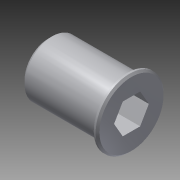
# Autodesk Inventor part: colson hub
Saved by Autodesk Inventor 2013 (Build 170138000, 138)
## iProperties
Created: 2012-09-06
Part Number: colson hub
Material: Aluminum 6061
Document SubType Name: Modeling
Designer: student
Density: 2.71 g/cm^3
Mass: 25.8237 g
Surface Area: 50.2015 cm^2
Volume: 9.52906 cm^3
Author: student
Autodesk Inventor part; units mm, degrees
ref_plane "YZ Plane" through (0, 0, 0) normal (1, 0, 0) x (0, 1, 0)
ref_plane "XZ Plane" through (0, 0, 0) normal (0, 1, 0) x (-1, 0, 0)
ref_plane "XY Plane" through (0, 0, 0) normal (0, 0, 1) x (1, 0, 0)
sketch "Sketch1" plane through (0, 0, 0) normal (1, 0, 0) x (0, 1, 0)
  circle A0 centre (0, 0) radius 11.684
  dimension "d0" = 23.368
  constraints: 1 centre point, 1 coincident
  measures "d0" diameter of A0
extrude "Extrusion1" add sketch "Sketch1" along normal blind 33.3375
sketch "Sketch2" plane through (33.3375, 0, 0) normal (1, 0, 0) x (0, 0, -1)
  circle A0 centre (0, 0) radius 11.684 projected
  circle A1 centre (0, 0) radius 14.2875
  dimension "d4" = 28.575
  constraints: 1 centre point, 1 coincident
  measures "d4" diameter of A1
extrude "Extrusion2" add sketch "Sketch2" along normal blind 1.5875 contours A0 | A1
sketch "Sketch3" plane through (34.925, 0, 0) normal (1, 0, 0) x (0, 0, -1)
  circle A0 centre (0, 0) radius 14.2875 projected
  line L0 (3.6662, 6.35) -> (7.3323, 0)
  line L1 (7.3323, 0) -> (3.6662, -6.35)
  line L2 (3.6662, -6.35) -> (-3.6662, -6.35)
  line L3 (-3.6662, -6.35) -> (-7.3323, 0)
  line L4 (-7.3323, 0) -> (-3.6662, 6.35)
  line L5 (-3.6662, 6.35) -> (3.6662, 6.35)
  dimension "d11" = 12.7
  constraints: 12 end point, 1 coincident, 1 horizontal, 13 other
  measures "d11" distance between parallel lines of L2 L5
extrude "Extrusion3" cut sketch "Sketch3" against normal blind 50.8 contours L0 L1 L2 L3 L4 L5
chamfer "Chamfer1" distance 0.7937 angle 45 1 edges at (34.925, 0, 14.2875)
chamfer "Chamfer2" distance 1.5875 angle 45 1 edges at (0, -11.684, 0)
body "Solid1"
